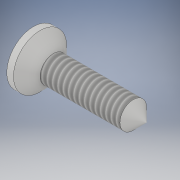
# Autodesk Inventor part: screw
Saved by Autodesk Inventor 2017.3 (Build 213256000, 256)
## iProperties
Created: 2017-04-21
Part Number: screw
Material: Generic
Document SubType Name: Modeling
Designer: 167898
Density: 1 g/cm^3
Appearance: Default
Author: 167898
Autodesk Inventor part; units mm, degrees
ref_plane "YZ Plane" through (0, 0, 0) normal (1, 0, 0) x (0, 1, 0)
ref_plane "XZ Plane" through (0, 0, 0) normal (0, 1, 0) x (-1, 0, 0)
ref_plane "XY Plane" through (0, 0, 0) normal (0, 0, 1) x (1, 0, 0)
sketch "Sketch1" plane through (0, 0, 0) normal (1, 0, 0) x (0, 1, 0)
  circle A0 centre (169.2255, 363.3555) radius 48.0965
  circle A1 centre (138.8493, 276.6293) radius 6.35
  point P0 (0, 0)
  dimension "d0" = 12.7
  constraints: 2 centre point
  measures "d0" diameter of A1
extrude "Extrusion1" add sketch "Sketch1" along normal blind 4.7625 contours A1
chamfer "Chamfer1" distance 3.175 angle 45 1 edges at (4.7625, 132.4993, 276.6293)
sketch "Sketch2" plane through (4.7625, 138.8493, 276.6293) normal (1, 0, 0) x (0, 0, -1)
  circle A0 centre (0, 0) radius 3.175 projected
  circle A1 centre (0, 0) radius 3.175
  point P0 (276.6293, -138.8493)
  constraints: 1 centre point, 1 coincident
extrude "Extrusion2" add sketch "Sketch2" along normal blind 22.225
chamfer "Chamfer2" distance 3.175 angle 45 1 edges at (26.9875, 138.8493, 279.8043)
sketch "Sketch3" plane through (0, 138.8493, 276.6293) normal (-1, 0, 0) x (0, 0, 1)
  point P0 (-276.6293, -138.8493)
thread "Thread1" size "1/4-20 UNC" class "2A" standard "ANSI Unified Screw Threads" full length
sketch "Sketch4" plane through (0, 138.8493, 276.6293) normal (-1, 0, 0) x (0, 0, 1)
  line L0 (-1.16, 5.6468) -> (1.058, 5.6468)
  line L1 (1.058, 5.6468) -> (1.058, -5.4225)
  line L2 (1.058, -5.4225) -> (-1.16, -5.4225)
  line L3 (-1.16, -5.4225) -> (-1.16, 5.6468)
  line L4 (-5.2022, 1.2937) -> (5.5977, 1.2937)
  line L5 (5.5977, 1.2937) -> (5.5977, -1.1109)
  line L6 (5.5977, -1.1109) -> (-5.2022, -1.1109)
  line L7 (-5.2022, -1.1109) -> (-5.2022, 1.2937)
  point P0 (-276.6293, -138.8493)
  constraints: 16 end point, 4 parallel, 2 horizontal, 2 perpendicular
extrude "Extrusion3" cut sketch "Sketch4" against normal blind 1.5875
body "Solid1"
